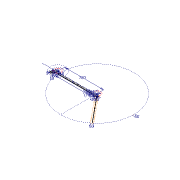
# Autodesk Inventor part: Soporte freno
Saved by Autodesk Inventor 2019 (Build 230136000, 136)
## iProperties
Created: 2020-02-07
Part Number: Soporte freno
Material: Generic
Document SubType Name: Modeling
Designer: Juan Carlos Botero
Density: 1 g/cm^3
Appearance: Default
Author: Juan Carlos Botero
Autodesk Inventor part; units mm, degrees
ref_plane "YZ Plane" through (0, 0, 0) normal (1, 0, 0) x (0, 1, 0)
ref_plane "XZ Plane" through (0, 0, 0) normal (0, 1, 0) x (-1, 0, 0)
ref_plane "XY Plane" through (0, 0, 0) normal (0, 0, 1) x (1, 0, 0)
sketch "Sketch1" plane through (0, 0, 0) normal (0, 1, 0) x (-1, 0, 0)
  line L0 (-32.0851, 0) -> (32.0851, 0)
  circle A0 centre (-707.9149, -25) radius 9.525 construction
  circle A1 centre (-708.1649, 701) radius 16.5354 construction
  line L1 (-708.1649, 701) -> (-707.9149, -25) construction
  line L2 (-707.9149, -25) -> (-1167.5404, 536.979)
  circle A2 centre (-707.9149, -25) radius 726 construction
  line L3 (-727.2668, -40.8273) -> (-1186.8923, 521.1517) construction
  line L4 (-1186.8923, 521.1517) -> (-1148.1885, 552.8064) construction
  line L5 (-1148.1885, 552.8064) -> (-688.563, -9.1727) construction
  line L6 (-688.563, -9.1727) -> (-727.2668, -40.8273) construction
  line L7 (-727.2668, -40.8273) -> (-1148.1885, 552.8064) construction
  line L8 (-1186.8923, 521.1517) -> (-688.563, -9.1727) construction
  line L9 (-1433.9063, -50.25) -> (-1433.9235, -0.25) construction
  line L10 (-707.9235, 0) -> (-707.9063, -50) construction
  circle A3 centre (-707.9149, -25) radius 52.5 construction
  line L11 (-697.3638, 39.6777) -> (-709.1385, 15.9848)
  line L12 (-708.9043, 53.7882) -> (-734.4622, 46.9478)
  arc A4 (-697.3638, 39.6777) -> (-708.9043, 53.7882) centre (-706.3189, 44.1282) ccw
  circle A5 centre (-706.3189, 44.1282) radius 5
  line L13 (-706.3189, 44.1282) -> (-741.1523, 15.639) construction
  circle A6 centre (72.0851, -25) radius 5
  arc A7 (62.8991, -21.0481) -> (80.3122, -19.3154) centre (72.0851, -25) ccw
  circle A8 centre (72.0851, -25) radius 87.2511 construction
  line L14 (176.9747, 84.4532) -> (127.3309, 55.4404) construction
  circle A9 centre (72.0851, -25) radius 151.5976 construction
  circle A10 centre (-707.9149, -25) radius 69.1466 construction
  line L15 (-707.9387, 44.1466) -> (-777.0615, -25) construction
  line L16 (80.7183, 20.3721) -> (62.8991, -21.0481)
  line L17 (-707.933, 27.5) -> (-662.933, 27.5155) construction
  circle A11 centre (72.0851, -25) radius 52.5 construction
  circle A12 centre (72.0851, -25) radius 69.1466 construction
  line L18 (72.0851, 27.5) -> (117.0851, 27.5) construction
  circle A13 centre (117.0851, 27.5) radius 5
  arc A14 (125.2839, 58.4267) -> (124.0817, 53.8433) centre (123.911, 56.3374) ccw
  line L19 (148.823, 13.7104) -> (125.945, 52.8571)
  arc A15 (125.2839, 58.4267) -> (127.3914, 58.3714) centre (126.3822, 60.0981) ccw
  arc A16 (125.945, 52.8571) -> (124.0817, 53.8433) centre (124.2183, 51.8479) ccw
  line L20 (-709.1385, 15.9848) -> (-734.4622, 46.9478)
  line L21 (148.823, 13.7104) -> (128.5153, 13.7104)
  line L22 (121.3974, 10.7344) -> (79.203, -32.024)
  arc A17 (128.5153, 13.7104) -> (121.3974, 10.7344) centre (128.5153, 3.7104) ccw
  line L23 (123.911, 56.3374) -> (175.7133, 86.6116) construction
  line L24 (154.1852, 4.5352) -> (123.911, 56.3374) construction
  line L25 (117.0851, 27.5) -> (-662.933, 27.5155) construction
  line L26 (117.0853, 37.5) -> (-662.9328, 37.5155) construction
  line L27 (-662.9332, 17.5155) -> (117.0849, 17.5) construction
  arc A18 (117.0849, 17.5) -> (117.0853, 37.5) centre (117.0851, 27.5) ccw construction
  arc A19 (-662.9328, 37.5155) -> (-662.9332, 17.5155) centre (-662.933, 27.5155) ccw construction
  line L28 (-732.9149, -5) -> (367.0851, -5) construction
  line L29 (-732.9149, 0) -> (367.0851, 0) construction
  line L30 (-760.4149, -25) -> (-760.4149, 20) construction
  line L31 (19.5851, -25) -> (19.5851, 20) construction
  line L32 (19.5851, 20) -> (-760.4149, 20) construction
  line L33 (19.5851, 30) -> (-760.4149, 30)
  line L34 (-760.4149, 10) -> (19.5851, 10)
  arc A20 (19.5851, 10) -> (19.5851, 30) centre (19.5851, 20) ccw
  arc A21 (-760.4149, 30) -> (-760.4149, 10) centre (-760.4149, 20) ccw
  line L35 (146.4702, 69.5214) -> (102.7028, 71.4745) construction
  line L36 (102.7028, 71.4745) -> (80.7183, 20.3721) construction
  spline S0 degree 2 poles (146.4702, 69.5214) (102.7028, 71.4745) (80.7183, 20.3721) knots 1 1 1 2 2 2
  line L37 (127.3914, 58.3714) -> (146.4702, 69.5214)
  circle A22 centre (19.5851, 20) radius 5
  circle A23 centre (-760.4149, 20) radius 5
  point P0 (0, 0)
  point P1 (0, 0)
  point P2 (-937.7276, 255.9895)
  point P3 (-707.9149, -25)
  point P4 (126.0694, 57.5988)
  point P5 (130.1781, 60)
  point P6 (125.1724, 54.179)
  point P7 (132.8635, 61.5694)
  point P8 (-272.9239, 27.5077)
  point P9 (-370.4149, 20)
  dimension "d8" = 50
  dimension "d9" = 50
  dimension "d10" = 105
  dimension "d13" = 10
  dimension "d14" = 20
  dimension "d15" = 20
  dimension "d16" = 40
  dimension "d17" = 10
  dimension "d18" = 780
  dimension "d19" = 20
  dimension "d23" = 45
  dimension "d24" = 10
  dimension "d26" = 5
  dimension "d27" = 2
  dimension "d28" = 45
  dimension "d31" = 69.147
  dimension "d32" = 10
  dimension "d33" = 20
  dimension "d34" = 20
  dimension "d35" = 780
  dimension "d36" = 10
  dimension "d37" = 10
  constraints: 76 end point, 37 point on circle, 22 centre point, 20 tangent, 15 coincident, 11 point on line, 8 midpoint, 6 parallel, 5 horizontal, 4 perpendicular, 3 equal radius, 2 vertical, 1 collinear, 1 equal length, 1 horizontal alignment, 27 other
  measures "d8" distance of L3.end L4.end
  measures "d9" distance of L9.start L9.end
  measures "d10" diameter of A3
  measures "d13" diameter of A5
  measures "d14" diameter of A4
  measures "d15" distance from line of L5 A4.centre
  measures "d16" distance of L11.end L12.end
  measures "d17" diameter of A6
  measures "d18" distance of L1.end A6.centre
  measures "d19" diameter of A7
  measures "d23" distance of L17.start L17.end
  measures "d24" diameter of A13
  measures "d26" diameter of A14
  measures "d27" radius of A15
  measures "d28" distance of L18.start L18.end
  measures "d32" radius of A17
  measures "d33" diameter of A19
  measures "d34" diameter of A21
  measures "d35" distance of L31.end L30.end
  measures "d36" diameter of A22
  measures "d37" diameter of A23
extrude "Extrusion1" add sketch "Sketch1" along normal mid plane 6 contours L16 S0 L37 A15 A14 A16 L19 L21 A17 L22 A7
extrude "Extrusion3" add sketch "Sketch1" along normal blind 6 separate body contours L33 L11 L20 | L20 L12 A4 L11 L33
extrude "Extrusion4" add sketch "Sketch1" along normal blind 6 separate body contours L34 A21 L33 L2 | L2 L33 L20 L11 A20 L34 | L33 L11 L20
sketch "Sketch3" plane through (0, -3, 0) normal (0, -1, 0) x (1, 0, 0)
  circle A0 centre (-118.8299, 37.0538) radius 5 projected
  circle A1 centre (-72.2906, -14.0866) radius 5 projected
  line L0 (-63.226, -9.8637) -> (-82.2675, 31.0091) projected
  spline S0 degree 2 poles (-82.2675, 31.0091) (-105.7599, 81.436) (-149.45, 78.184) knots 1 1 1 2 2 2 projected
  line L1 (-149.45, 78.184) -> (-130.0484, 67.6055) projected
  arc A2 (-130.0484, 67.6055) -> (-127.9435, 67.7234) centre (-129.091, 69.3615) ccw projected
  arc A3 (-126.6058, 63.1776) -> (-127.9435, 67.7234) centre (-126.5092, 65.6758) ccw projected
  arc A4 (-126.6058, 63.1776) -> (-128.4389, 62.1366) centre (-126.683, 61.1791) ccw projected
  line L2 (-128.4389, 62.1366) -> (-150.1443, 22.3278) projected
  line L3 (-150.1443, 22.3278) -> (-129.8455, 22.9309) projected
  arc A5 (-122.6424, 20.1675) -> (-129.8455, 22.9309) centre (-129.5485, 12.9353) ccw projected
  line L4 (-122.6424, 20.1675) -> (-79.1967, -21.3189) projected
  arc A6 (-79.1967, -21.3189) -> (-63.226, -9.8637) centre (-72.2906, -14.0866) ccw projected
  arc A7 (-125.4874, 22.0735) -> (-102.6507, 39.693) centre (-118.8299, 37.0538) ccw
  line L5 (-149.45, 78.184) -> (-109.6014, 82.3028) construction
  line L6 (-109.6014, 82.3028) -> (-102.6507, 39.693) construction
  spline S1 degree 2 poles (-149.45, 78.184) (-109.6014, 82.3028) (-102.6507, 39.693) knots 1 1 1 2 2 2
  point P0 (0, 0)
  constraints: 3 point on circle, 2 tangent, 1 centre point, 1 coincident, 3 other
extrude "Extrusion5" add sketch "Sketch3" along normal blind 6 separate body contours S1 A7 A5 L3 L2 A4 A3 A2 L1 S0 | S0 S1
body "Solid1"
body "Solid2"
